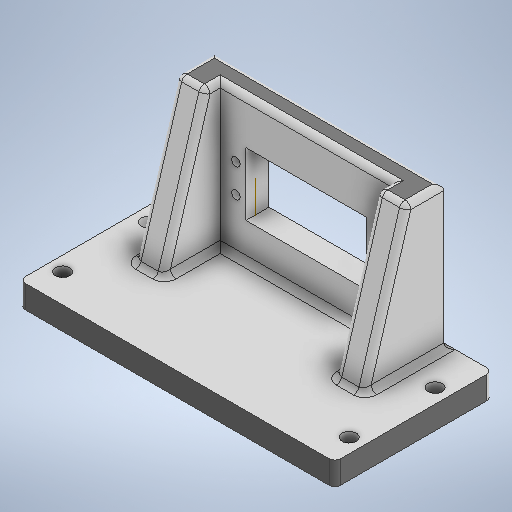
# Autodesk Inventor part: MG996R_PODSTAWA
Saved by Autodesk Inventor 2025.2 (Build 292293000, 293)
## iProperties
Created: 2025-11-25
Part Number: MG996R_PODSTAWA
Material: Ogólny
Document SubType Name: Modeling
Designer: juras
Density: 1 g/cm^3
Appearance: Domyślna
Author: juras
Autodesk Inventor part; units mm, degrees
ref_plane "YZ Plane" through (0, 0, 0) normal (1, 0, 0) x (0, 1, 0)
ref_plane "XZ Plane" through (0, 0, 0) normal (0, 1, 0) x (-1, 0, 0)
ref_plane "XY Plane" through (0, 0, 0) normal (0, 0, 1) x (1, 0, 0)
sketch "Szkic1" plane through (0, 0, 0) normal (0, 1, 0) x (-1, 0, 0)
  line L0 (55, 45) -> (-55, 45)
  line L1 (-55, 45) -> (-55, -45)
  line L2 (-55, -45) -> (55, -45)
  line L3 (55, -45) -> (55, 45)
  line L4 (55, 45) -> (-55, -45) construction
  line L5 (-55, 45) -> (55, -45) construction
  point P0 (0, 0)
  dimension "d0" = 110
  dimension "d1" = 90
  constraints: 12 end point, 2 midpoint, 2 parallel, 1 horizontal, 1 perpendicular
  measures "d0" distance of L2.end L1.end
  measures "d1" distance of L1.end L0.end
extrude "Wyciągnięcie proste1" add sketch "Szkic1" along normal mid plane 8
fillet "Zaokrąglenie1" radius 2 4 edges at (-55, 0, -45) (-55, 0, 45) (55, 0, 45) (55, 0, -45)
sketch "Szkic5" plane through (0, 4, 0) normal (0, 1, 0) x (1, 0, 0)
  line L0 (0, 0) -> (22, 0)
  line L1 (0, 0) -> (-22, 0)
  line L2 (-22, 0) -> (-32, 0)
  line L3 (-32, 0) -> (-32, -20)
  line L4 (-32, -20) -> (-22, -20)
  line L5 (-22, -20) -> (-22, 0)
  line L6 (22, 0) -> (32, 0)
  line L7 (32, 0) -> (32, -20)
  line L8 (32, -20) -> (22, -20)
  line L9 (22, -20) -> (22, 0)
  line L10 (-32, 0) -> (32, 0)
  line L11 (32, 0) -> (32, 8)
  line L12 (32, 8) -> (-32, 8)
  line L13 (-32, 8) -> (-32, 0)
  point P0 (32, 0)
  dimension "d14" = 22
  dimension "d15" = 22
  dimension "d16" = 10
  dimension "d17" = 20
  dimension "d18" = 10
  dimension "d19" = 20
  dimension "d20" = 64
  dimension "d21" = 8
  constraints: 28 end point, 6 parallel, 5 horizontal, 3 perpendicular
  measures "d14" distance of L0.start L0.end
  measures "d15" distance of L0.start L1.end
  measures "d16" distance of L4.end L3.end
  measures "d17" distance of L3.end L2.end
  measures "d18" distance of L7.end L8.end
  measures "d19" distance of L6.end L7.end
  measures "d20" distance of L12.end L11.end
  measures "d21" distance of L11.end L10.end
extrude "Wyciągnięcie proste2" add sketch "Szkic5" along normal blind 50
sketch "Szkic8" plane through (-22, 4, 0) normal (0, 0, 1) x (1, 0, 0)
  point P0 (22, -4)
sketch "Szkic10" plane through (-22, 4, 0) normal (0, 0, 1) x (1, 0, 0)
  point P0 (22, -4)
sketch "Szkic13" plane through (-22, 4, 20) normal (1, 0, 0) x (0, 0, -1)
  line L0 (0, 50) -> (20, 50) projected
  line L1 (20, 50) -> (0, 0)
  line L2 (0, 0) -> (0, 50) projected
  line L3 (0, 0) -> (0, 50)
  line L4 (0, 50) -> (20, 50)
  point P0 (20, -4)
  constraints: 6 end point, 1 collinear, 1 perpendicular, 1 point on line
extrude "Wyciągnięcie proste4" cut sketch "Szkic13" against normal blind 20
sketch "Szkic14" plane through (22, 4, 0) normal (-1, 0, 0) x (0, 0, 1)
  line L0 (0, 50) -> (20, 50) projected
  line L1 (0, 50) -> (20, 50)
  line L2 (20, 0) -> (0, 0) projected
  line L3 (20, 50) -> (20, 0)
  line L4 (0, 0) -> (0, 50) projected
  line L5 (20, 0) -> (0, 50)
  point P0 (0, -4)
  point P1 (0, 36)
  constraints: 6 end point, 1 collinear, 1 perpendicular
extrude "Wyciągnięcie proste5" cut sketch "Szkic14" against normal blind 25 contours L0 L3 L5
fillet "Zaokrąglenie2" radius 2 6 edges at (-32, 29, -8) (-32, 29, 10) (-22, 29, 10) (22, 29, 10) (32, 29, 10) (32, 29, -8)
sketch "Szkic15" plane through (-32, 4, -6) normal (-1, 0, 0) x (0, 0, 1)
  point P0 (6, -4)
sketch "Szkic18" plane through (0, 4, 0) normal (0, 1, 0) x (1, 0, 0)
  point P0 (0, 0)
sketch "Szkic20" plane through (0, 4, 0) normal (0, 1, 0) x (1, 0, 0)
  line L0 (50, -5) -> (-50, -5)
  line L1 (-50, -5) -> (-50, -40)
  line L2 (-50, -40) -> (50, -40)
  line L3 (50, -40) -> (50, -5)
  line L4 (55, -43) -> (55, 43) projected
  line L5 (40, 0) -> (17, 0) projected
  line L6 (-55, 43) -> (-55, -43) projected
  line L7 (-53, -45) -> (53, -45) projected
  point P0 (0, 0)
  point P1 (26, 10)
  point P2 (-30, 10)
  point P3 (-55, -43)
  dimension "d73" = 5
  dimension "d75" = 5
  dimension "d76" = 5
  dimension "d90" = 40
  constraints: 8 end point, 2 parallel, 1 horizontal, 1 perpendicular, 3 other
  measures "d76" distance between parallel lines of L7 L2
  measures "d90" distance from line of L7 L0.start
hole "Otwór4" at (50, 4, 5) at (-50, 4, 5) direction (0, -1, 0) diameter 5 end through all
sketch "Szkic22" plane through (0, 4, 0) normal (0, 1, 0) x (1, 0, 0)
  circle A0 centre (-50, -35) radius 2.5
  line L0 (-55, 43) -> (-55, -43) projected
  line L1 (-53, -45) -> (53, -45) projected
  point P0 (0, 0)
  point P1 (-40, 10)
  point P2 (-55, -43)
  dimension "d91" = 5
  dimension "d92" = 5
  dimension "d93" = 10
  constraints: 1 centre point, 1 other
  measures "d91" diameter of A0
  measures "d93" distance from line of A0.centre L1
extrude "Wyciągnięcie proste10" cut sketch "Szkic22" against normal blind 10
mirror "Odbij1" about plane through (0, 0, 0) normal (1, 0, 0) of "Wyciągnięcie proste10"
sketch "Szkic23" plane through (0, 4, 0) normal (0, 1, 0) x (1, 0, 0)
  line L0 (-55, 43) -> (-55, -43) projected
  line L1 (55, 45) -> (-55, 45)
  line L2 (-55, 45) -> (-55, 10)
  line L3 (-55, 10) -> (55, 10)
  line L4 (55, 10) -> (55, 45)
  line L5 (-53, -45) -> (53, -45) projected
  point P0 (0, 0)
  dimension "d97" = 55
  dimension "d98" = 110
  dimension "d99" = 90
  constraints: 8 end point, 2 parallel, 1 horizontal, 1 perpendicular, 1 point on line
  measures "d97" distance between parallel lines of L3 L5
  measures "d98" distance between parallel lines of L0 L4
  measures "d99" distance between parallel lines of L5 L1
extrude "Wyciągnięcie proste11" cut sketch "Szkic23" against normal blind 10
fillet "Zaokrąglenie4" radius 2 2 edges at (55, 0, -10) (-55, 0, -10)
sketch "Szkic24" plane through (30, 54, -8) normal (0, 0, -1) x (-1, 0, 0)
  circle A0 centre (54.5, -21.5) radius 1.5
  line L0 (52, -14) -> (52, -36) projected
  line L1 (8, -14) -> (51, -14) projected
  circle A1 centre (5.5, -31.5) radius 1.5
  line L2 (8, -36) -> (8, -14) projected
  circle A2 centre (54.5, -31.5) radius 1.5
  line L3 (8, -36) -> (8, -14) projected
  line L4 (0, 0) -> (60, 0) projected
  point P0 (30, -54)
  dimension "d104" = 3
  dimension "d105" = 2.5
  dimension "d109" = 7.5
  dimension "d113" = 3
  dimension "d114" = 10
  dimension "d115" = 2.5
  dimension "d135" = 49
  dimension "d136" = 3
  dimension "d137" = 31.5
  constraints: 3 centre point
  measures "d104" diameter of A0
  measures "d105" distance from line of A0.centre L0
  measures "d109" distance from line of L1 A0.centre
  measures "d113" diameter of A2
  measures "d114" distance of A2.centre A0.centre
  measures "d115" distance from line of A2.centre L0
  measures "d135" distance of A2.centre A1.centre
  measures "d136" diameter of A1
  measures "d137" distance from line of L4 A1.centre
extrude "Wyciągnięcie proste12" cut sketch "Szkic24" against normal blind 15
ref_plane "Płaszczyzna konstrukcyjna1" through (-32, 16.5, -3.2446) normal (0, 0, 1) x (1, 0, 0)
sketch "Szkic25" plane through (-32, 16.5, -3.2446) normal (0, 0, 1) x (1, 0, 0)
  line L0 (11, 0) -> (53, 0)
  line L1 (53, 0) -> (53, 22)
  line L2 (53, 22) -> (11, 22)
  line L3 (11, 22) -> (11, 0)
  line L4 (11, 0) -> (53, 22) construction
  line L5 (53, 0) -> (11, 22) construction
  line L6 (8, 36) -> (56, 36) projected
  line L7 (11, -14) -> (53, -14) projected
  line L8 (10, 0) -> (10, 20.4112) projected
  line L9 (54, 30.6148) -> (54, -14) projected
  point P0 (32, -16.5)
  point P1 (32, 11)
  point P2 (54, -13)
  dimension "d125" = 14
  dimension "d126" = 14
  dimension "d127" = 1
  dimension "d128" = 1
  constraints: 12 end point, 2 midpoint, 2 parallel, 1 horizontal, 1 perpendicular
  measures "d125" distance between parallel lines of L2 L6
  measures "d126" distance between parallel lines of L7 L0
  measures "d127" distance between parallel lines of L8 L3
  measures "d128" distance between parallel lines of L9 L1
extrude "Wyciągnięcie proste13" cut sketch "Szkic25" against normal blind 10
sketch "Szkic26" plane through (30, 54, -8) normal (0, 0, -1) x (-1, 0, 0)
  circle A0 centre (5.5, -21.5) radius 1.5
  circle A1 centre (5.5, -31.5) radius 1.5 projected
  circle A2 centre (54.5, -21.5) radius 1.5 projected
  point P0 (30, -54)
  dimension "d131" = 3
  dimension "d132" = 10
  dimension "d133" = 49
  constraints: 1 centre point
  measures "d131" diameter of A0
  measures "d132" distance of A0.centre A1.centre
  measures "d133" distance of A0.centre A2.centre
extrude "Wyciągnięcie proste14" cut sketch "Szkic26" against normal blind 15 contours A0
sketch "Szkic27" plane through (0, 4, 0) normal (0, 1, 0) x (1, 0, 0)
  point P0 (0, 0)
sketch "Szkic28" plane through (0, 4, 0) normal (0, 1, 0) x (1, 0, 0)
  line L0 (-30, 8) -> (30, 8) projected
  line L1 (-30, 8) -> (-40, 8)
  line L2 (-40, 8) -> (-40, -20)
  line L3 (-40, -20) -> (-30, -20)
  line L4 (-30, -20) -> (-30, 8)
  point P0 (0, 0)
  dimension "d140" = 10
  dimension "d141" = 28
  constraints: 8 end point, 2 parallel, 1 horizontal, 1 perpendicular
  measures "d140" distance of L3.end L2.end
  measures "d141" distance of L2.end L1.end
extrude "Wyciągnięcie proste15" add sketch "Szkic28" along normal blind 50
sketch "Szkic29" plane through (-32, 16.5, -3.2446) normal (0, 0, -1) x (-1, 0, 0)
  line L0 (-11, 0) -> (-53, 0) projected
  line L1 (-53, 22) -> (-11, 22) projected
  line L2 (-53, 0) -> (-11, 0)
  line L3 (-11, 0) -> (-11, 22)
  line L4 (-11, 22) -> (-53, 22)
  line L5 (-53, 22) -> (-53, 0)
  point P0 (-32, -16.5)
  constraints: 8 end point, 2 parallel, 1 horizontal, 1 perpendicular
extrude "Wyciągnięcie proste16" cut sketch "Szkic29" against normal blind 15
sketch "Szkic30" plane through (0, 4, 0) normal (0, 1, 0) x (1, 0, 0)
  line L0 (-30, -20) -> (-40, -20) projected
  line L1 (22, 0) -> (-22, 0) projected
  line L2 (-30, -20) -> (-22, -20)
  line L3 (-22, -20) -> (-22, 0)
  line L4 (-22, 0) -> (-30, 0)
  line L5 (-30, 0) -> (-30, -20)
  point P0 (0, 0)
  constraints: 8 end point, 2 parallel, 1 horizontal, 1 perpendicular
extrude "Wyciągnięcie proste17" cut sketch "Szkic30" along normal blind 155
sketch "Szkic31" plane through (-30, 4, 20) normal (1, 0, 0) x (0, 0, -1)
  line L0 (0, 50) -> (20, 50) projected
  line L1 (0, 50) -> (15, 50)
  line L2 (28, 50) -> (0, 50) projected
  line L3 (0, 0) -> (0, 50) projected
  line L4 (15, 50) -> (0, 0)
  line L5 (0, 0) -> (0, 50)
  point P0 (20, -4)
  dimension "d148" = 15
  constraints: 6 end point, 1 collinear, 1 point on line
  measures "d148" distance of L0.start L1.end
extrude "Wyciągnięcie proste18" cut sketch "Szkic31" against normal blind 155
sketch "Szkic32" plane through (0, 4, 0) normal (0, 1, 0) x (1, 0, 0)
  arc A0 (32, 6) -> (30, 8) centre (30, 6) ccw projected
  line L0 (30, 8) -> (40, 8)
  line L1 (40, 8) -> (40, -20)
  line L2 (40, -20) -> (30, -20)
  line L3 (30, -20) -> (30, 8)
  point P0 (0, 0)
  dimension "d151" = 10
  dimension "d152" = 28
  constraints: 8 end point, 2 parallel, 1 horizontal, 1 perpendicular
  measures "d151" distance of L1.end L2.end
  measures "d152" distance of L0.end L1.end
extrude "Wyciągnięcie proste19" add sketch "Szkic32" along normal blind 50
sketch "Szkic33" plane through (0, 4, 0) normal (0, 1, 0) x (1, 0, 0)
  line L0 (22, -17.8459) -> (22, 0) projected
  line L1 (40, -20) -> (30, -20) projected
  line L2 (22, 0) -> (30, 0)
  line L3 (30, 0) -> (30, -20)
  line L4 (30, -20) -> (22, -20)
  line L5 (22, -20) -> (22, 0)
  point P0 (0, 0)
  point P1 (22, -17.8459)
  constraints: 8 end point, 2 parallel, 1 horizontal, 1 perpendicular
extrude "Wyciągnięcie proste20" cut sketch "Szkic33" along normal blind 55
mirror "Odbij5" about plane through (0, 0, 0) normal (1, 0, 0) of "Wyciągnięcie proste18"
fillet "Zaokrąglenie6" radius 2 20 edges at (0, 4, 0) (-30, 4, 10) (0, 4, -8) (-40, 4, 6) (-35, 4, 20) (35, 4, 20) (30, 4, 10) (40, 4, 6) (-30, 29, 12.5) (-40, 29, 12.5) (-35, 54, 5) (35, 54, 5) (30, 29, 12.5) (40, 29, 12.5) (0, 54, 0) (30, 54, 2.5) (0, 54, -8) (40, 54, -1.5) (-40, 54, -1.5) (-30, 54, 2.5)
